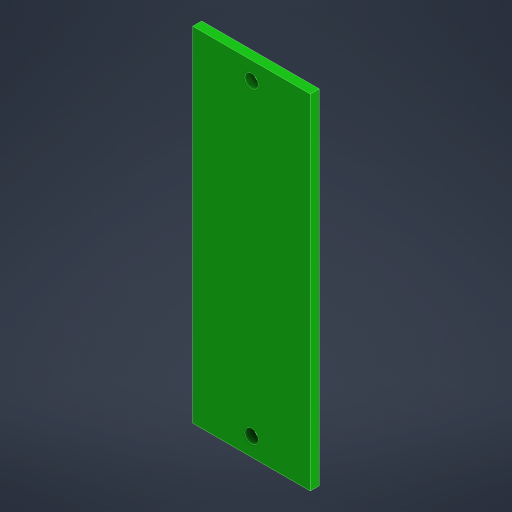
# Autodesk Inventor part: płytka_pcb
Saved by Autodesk Inventor 2023.4 (Build 274418000, 418)
## iProperties
Created: 2025-10-31
Part Number: płytka_pcb
Material: Tworzywo sztuczne ABS
Document SubType Name: Modeling
Designer: Jakub Borsukiewicz
Density: 1.06 g/cm^3
Appearance: Ciemnozielona
Author: Jakub Borsukiewicz
Autodesk Inventor part; units mm, degrees
ref_plane "YZ Plane" through (0, 0, 0) normal (1, 0, 0) x (0, 1, 0)
ref_plane "XZ Plane" through (0, 0, 0) normal (0, 1, 0) x (-1, 0, 0)
ref_plane "XY Plane" through (0, 0, 0) normal (0, 0, 1) x (1, 0, 0)
sketch "Szkic1" plane through (0, 0, 0) normal (0, 0, 1) x (1, 0, 0)
  line L0 (0, -7.6) -> (0, 45.6) projected
  line L1 (-5.2, 0) -> (31.2, 0) projected
  line L2 (0, 0) -> (26, 0)
  line L3 (26, 0) -> (26, 38)
  line L4 (26, 38) -> (0, 38)
  line L5 (0, 38) -> (0, 0)
  circle A0 centre (13, 34) radius 1.5
  point P0 (0, 38)
  dimension "d0" = 26
  dimension "d1" = 38
  dimension "d2" = 3
  dimension "d3" = 4
  dimension "d4" = 13
  constraints: 8 end point, 2 parallel, 1 centre point, 1 horizontal, 1 perpendicular
  measures "d0" distance of L3.end L4.end
  measures "d1" distance of L2.end L3.end
  measures "d2" diameter of A0
  measures "d3" distance from line of L4 A0.centre
  measures "d4" distance from line of L5 A0.centre
extrude "Wyciągnięcie proste1" add sketch "Szkic1" along normal blind 2
mirror "Odbij1" about plane through (0, 0, 0) normal (0, 1, 0) of "Wyciągnięcie proste1"
